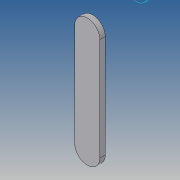
# Autodesk Inventor part: Batterycase_deckel
Saved by Autodesk Inventor 2019.4 (Build 234330000, 330)
## iProperties
Part Number: Batterycase_deckel
Material: GEDA Stahl
Document SubType Name: Modeling
Designer: Admin
Mass: 25.7604 g
Surface Area: 34.0927 cm^2
Volume: 3.2774 cm^3
Density: 7.86 g/cm^3
Appearance: GEDA Stahl A
Author: Admin
Gewicht: 0,026 kg
G_L: 0
G_H: 0
G_B: 0
InventorVersion: 2019.4
VAULT_Status: in Bearbeitung
Revision: -
Max. Breite: 0
Max. Höhe: 0
Max. Länge: 0
Max. Abmessungen: 0 x 0 x 0
Autodesk Inventor part; units mm, degrees
note: some values were not read from the file. Left out: dimensions or parameters whose unit could not be read.
ref_plane "YZ Plane" through (0, 0, 0) normal (1, 0, 0) x (0, 1, 0)
ref_plane "XZ Plane" through (0, 0, 0) normal (0, 1, 0) x (-1, 0, 0)
ref_plane "XY Plane" through (0, 0, 0) normal (0, 0, 1) x (1, 0, 0)
sketch "Skizze1" plane through (0, 0, 0) normal (0, 1, 0) x (-1, 0, 0)
  line L0 (0, 19) -> (0, -19) construction
  line L1 (-9.3, 19) -> (-9.3, -19)
  line L2 (9.3, -19) -> (9.3, 19)
  arc A0 (9.3, 19) -> (-9.3, 19) centre (0, 19) ccw
  arc A1 (-9.3, -19) -> (9.3, -19) centre (0, -19) ccw
  line L3 (0, 19) -> (0, -19) construction
  line L4 (-10.8, 19) -> (-10.8, -19)
  line L5 (10.8, -19) -> (10.8, 19)
  arc A2 (10.8, 19) -> (-10.8, 19) centre (0, 19) ccw
  arc A3 (-10.8, -19) -> (10.8, -19) centre (0, -19) ccw
  point P0 (0, 0)
  dimension "d0" = 19
  dimension "d1" = 18.6
  dimension "d2" = 1.5
  constraints: 16 end point, 8 point on circle, 8 tangent, 4 centre point, 3 parallel, 2 midpoint, 1 vertical
  measures "d0" distance of point (0, 0) L0.end
  measures "d1" diameter of A1
  measures "d2" distance between parallel lines of L5 L2
extrude "Extrusion1" add sketch "Skizze1" along normal blind 4 contours A0 L2 A1 L1
extrude "Extrusion2" add sketch "Skizze1" against normal blind 2 contours A0 L2 A1 L1 | A2 L5 A3 L4
fillet "Rundung1" radius 2 4 edges at (-10.8, -2, 0) (0, -2, -29.8) (10.8, -2, 0) (0, -2, 29.8)
sketch "Skizze2" plane through (0, 4, 0) normal (0, 1, 0) x (1, 0, 0)
  line L0 (0, -19) -> (0, 19) construction
  line L1 (-7.3, -19) -> (-7.3, 19)
  line L2 (7.3, 19) -> (7.3, -19)
  arc A0 (-7.3, -19) -> (7.3, -19) centre (0, -19) ccw
  arc A1 (7.3, 19) -> (-7.3, 19) centre (0, 19) ccw
  arc A2 (9.3, 19) -> (-9.3, 19) centre (0, 19) ccw projected
  line L3 (9.3, -19) -> (9.3, 19) projected
  point P0 (0, 0)
  dimension "d8" = 2
  constraints: 8 end point, 4 point on circle, 4 tangent, 2 centre point, 1 concentric, 1 midpoint, 1 parallel, 1 vertical
  measures "d8" distance between parallel lines of L3 L2
extrude "Extrusion3" cut sketch "Skizze2" against normal blind 4
fillet "Rundung2" radius 2 4 edges at (0, 0, 26.3) (-7.3, 0, 0) (0, 0, -26.3) (7.3, 0, 0)
sketch "Skizze3" plane through (0, 0, 0) normal (0, 1, 0) x (1, 0, 0)
  circle A0 centre (3.3, 10) radius 4
  line L0 (7.3, 19) -> (7.3, -19) projected
  point P0 (0, 0)
  dimension "d12" = 8
  dimension "d13" = 10
  constraints: 1 centre point, 1 tangent
  measures "d12" diameter of A0
  measures "d13" vertical distance of point (0, 0) A0.centre
extrude "Extrusion4" cut sketch "Skizze3" along normal mid plane 4
equation "\"G_L\" = 0"
equation "\"G_H\" = 0"
equation "\"G_B\" = 0"
